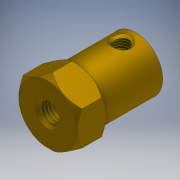
# Autodesk Inventor part: 6mmID_30mmL_hex_adapter
Saved by Autodesk Inventor 2018 (Build 220112000, 112)
## iProperties
Created: 2019-05-08
Part Number: 6mmID_30mmL_hex_adapter
Material: Generic
Document SubType Name: Modeling
Designer: ZEUSLAP
Density: 1 g/cm^3
Appearance: Default
Author: ZEUSLAP
Autodesk Inventor part; units mm, degrees
ref_plane "YZ Plane" through (0, 0, 0) normal (1, 0, 0) x (0, 1, 0)
ref_plane "XZ Plane" through (0, 0, 0) normal (0, 1, 0) x (-1, 0, 0)
ref_plane "XY Plane" through (0, 0, 0) normal (0, 0, 1) x (1, 0, 0)
sketch "Sketch1" plane through (0, 0, 0) normal (0, 1, 0) x (-1, 0, 0)
  line L0 (6, -3.4641) -> (0, -6.9282)
  line L1 (0, -6.9282) -> (-6, -3.4641)
  line L2 (-6, -3.4641) -> (-6, 3.4641)
  line L3 (-6, 3.4641) -> (0, 6.9282)
  line L4 (0, 6.9282) -> (6, 3.4641)
  line L5 (6, 3.4641) -> (6, -3.4641)
  circle A0 centre (0, 0) radius 2
  dimension "d0" = 6
  dimension "d1" = 4
  constraints: 12 end point, 2 coincident, 1 centre point, 13 other
  measures "d0" distance from line of L5 point (0, 0)
  measures "d1" diameter of A0
extrude "Extrusion1" add sketch "Sketch1" along normal blind 6
sketch "Sketch2" plane through (0, 6, 0) normal (0, 1, 0) x (1, 0, 0)
  circle A0 centre (0, 0) radius 3
  circle A1 centre (0, 0) radius 5.5
  dimension "d4" = 6
  dimension "d5" = 11
  constraints: 2 centre point, 2 coincident
  measures "d4" diameter of A0
  measures "d5" diameter of A1
extrude "Extrusion2" add sketch "Sketch2" along normal blind 12
sketch "Sketch3" plane through (0, 0, 0) normal (0, 0, 1) x (1, 0, 0)
  circle A0 centre (0, 15) radius 1.5
  line L0 (0, 0) -> (0, 6) projected
  line L1 (5.5, 18) -> (-5.5, 18) projected
  dimension "d16" = 3
  dimension "d44" = 0
  dimension "d45" = 3
  constraints: 1 centre point
  measures "d16" diameter of A0
  measures "d44" distance from line of L0 A0.centre
  measures "d45" distance from line of A0.centre L1
extrude "Extrusion3" cut sketch "Sketch3" along normal mid plane 24
chamfer "Chamfer" distance 0.5 angle 45 4 edges at (2, 0, 0) (-3, 18, 0) (-1.5, 15.0054, -5.2915) (-1.5, 15.0054, 5.2915)
sketch "Sketch4" plane through (0, 0, 0) normal (1, 0, 0) x (0, 1, 0)
  line L0 (0, -3.4641) -> (0, -6.9282) projected
  line L1 (0, -6.9282) -> (0, -5.9282)
  line L2 (0, -6.9282) -> (1, -6.9282)
  line L3 (1, -6.9282) -> (0, -5.9282)
  line L4 (-6, 0) -> (36, 0) projected
  line L5 (0, -6.9282) -> (6, -6.9282) projected
  line L6 (6, -6.9282) -> (5, -6.9282)
  line L7 (6, -6.9282) -> (6, -5.9282)
  line L8 (6, -5.9282) -> (5, -6.9282)
  dimension "d31" = 1
  dimension "d32" = 1
  dimension "d36" = 1
  dimension "d37" = 1
  constraints: 12 end point, 2 point on line, 1 horizontal, 1 perpendicular
  measures "d31" distance of L0.end L1.end
  measures "d32" distance of L0.end L2.end
  measures "d36" distance of L5.end L6.end
  measures "d37" distance of L5.end L7.end
revolve "Revolution" cut sketch "Sketch4" angle 360 about axis through (0, -10, 0) along (0, 1, 0)
thread "Thread1" size "M3x0.5" class "6H" standard "ANSI Metric M Profile" full length
thread "Thread2" size "M3x0.5" class "6H" standard "ANSI Metric M Profile" full length
thread "Thread3" size "M4x0.7" class "6H" standard "ANSI Metric M Profile" full length
body "Solid1"
